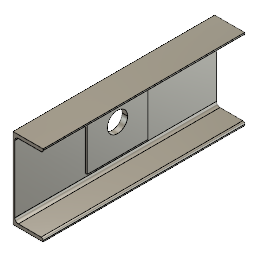
(25;;5@ 24_ version ECO (Autodesk Fusion 360 design; units mm, degrees)
Autodesk Fusion 360 part; units mm, degrees
sketch "Sketch1" plane through (0, 0, 0) normal (0, 0, 1) x (1, 0, 0)
  line L0 (0, 0) -> (0, 120)
  line L1 (0, 120) -> (90, 120)
  line L2 (5.6, 99.5) -> (5.6, 0)
  line L3 (90, 116) -> (90, 120)
  line L4 (0, 0) -> (5.6, 0)
  line L5 (16.1, 110) -> (84, 110)
  arc A0 (16.1, 110) -> (5.6, 99.5) centre (16.1, 99.5) ccw
  arc A1 (84, 110) -> (90, 116) centre (84, 116) ccw
  line L6 (0, -120) -> (90, -120)
  arc A2 (5.6, -99.5) -> (16.1, -110) centre (16.1, -99.5) ccw
  line L7 (90, -116) -> (90, -120)
  arc A3 (90, -116) -> (84, -110) centre (84, -116) ccw
  line L8 (16.1, -110) -> (84, -110)
  line L9 (0, 0) -> (0, -120)
  line L10 (5.6, -99.5) -> (5.6, 0)
  dimension "d3" = 120
  dimension "d4" = 90
  dimension "d5" = 5.6
  dimension "d8" = 10.5
  dimension "d9" = 6
  dimension "d10" = 10
  measures "d5" distance of L0.start
  measures "d8" radius of A0
  measures "d9" radius of A1
  measures "d10" distance of L1 L5
extrude "Extrude1" add sketch "Sketch1" along normal blind 600
sketch "Sketch2" plane through (0, 0, 0) normal (-1, 0, 0) x (0, 0, 1)
  line L0 (0, 120) -> (0, -120)
  line L1 (0, -120) -> (600, -120)
  line L2 (600, -120) -> (600, 120)
  line L3 (600, 120) -> (0, 120)
  circle A0 centre (300, 0) radius 30
  circle A1 centre (300, 0) radius 60
  dimension "d13" = 60
  dimension "d14" = 300
  dimension "d15" = 120
  dimension "d28" = 120
  measures "d13" diameter of A0
  measures "d15" distance of L3 origin
  measures "d28" diameter of A1
extrude "Extrude2" cut sketch "Sketch2" along normal through all and the other way blind 200 contours A0
sketch "Sketch6" plane through (0, 0, 0) normal (-1, 0, 0) x (0, 0, 1)
  circle A0 centre (300, 0) radius 30
  line L0 (0, 120) -> (0, -120)
  line L1 (0, -120) -> (600, -120)
  line L2 (600, -120) -> (600, 120)
  line L3 (600, 120) -> (0, 120)
  line L4 (210, 90) -> (390, 90)
  line L5 (390, 90) -> (390, -90)
  line L6 (390, -90) -> (210, -90)
  line L7 (210, -90) -> (210, 90)
  dimension "d41" = 180
  dimension "d42" = 180
  dimension "d43" = 90
  dimension "d44" = 90
  measures "d41" distance of origin
  measures "d43" distance of origin L4
  measures "d44" distance of origin L5
extrude "Extrude7" add sketch "Sketch6" along normal blind 5.6 contours L4 L5 L6 L7
sketch "Sketch7" plane through (5.6, 0, 0) normal (1, 0, 0) x (0, 0, -1)
  circle A0 centre (-300, 0) radius 30
  line L0 (0, -99.5) -> (0, 99.5)
  line L1 (0, 99.5) -> (-600, 99.5)
  line L2 (-600, 99.5) -> (-600, -99.5)
  line L3 (-600, -99.5) -> (0, -99.5)
  line L4 (-390, 90) -> (-210, 90)
  line L5 (-210, 90) -> (-210, -90)
  line L6 (-210, -90) -> (-390, -90)
  line L7 (-390, -90) -> (-390, 90)
  dimension "d47" = 180
  dimension "d48" = 180
  dimension "d49" = 90
  dimension "d50" = 90
  measures "d47" distance of origin
  measures "d49" distance of origin L6
extrude "Extrude8" add sketch "Sketch7" along normal blind 5.6 contours L4 L5 L6 L7
split_face "SplitFace3" 1 faces at (1.8667, 2.987, 329.8509) by plane through (0, 0, 0) normal (0, 1, 0)
equation "d3 = ( 240 / 2 ) * 1 mm"
